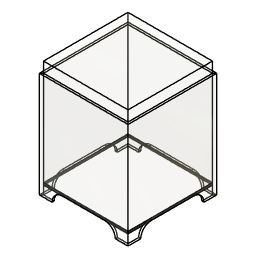
cube_fusion_model (Autodesk Fusion 360 design; units mm, degrees)
Autodesk Fusion 360 part; units mm, degrees
ref_plane "WorkPlane1" through (0, 0, 2) normal (0, 0, 1) x (1, 0, 0)
sketch "Sketch1" plane through (0, 0, 2) normal (0, 0, 1) x (1, 0, 0)
  line L0 (42.1, 42.1) -> (-42.1, 42.1)
  line L1 (-42.1, 42.1) -> (-42.1, -42.1)
  line L2 (-42.1, -42.1) -> (42.1, -42.1)
  line L3 (42.1, -42.1) -> (42.1, 42.1)
  line L4 (40, 40) -> (-40, 40)
  line L5 (-40, 40) -> (-40, -40)
  line L6 (-40, -40) -> (40, -40)
  line L7 (40, -40) -> (40, 40)
  line L8 (40, 40) -> (-40, -40) construction
  line L9 (-40, 40) -> (40, -40) construction
  line L10 (-40.1, 40.1) -> (-40.1, -40.1)
  line L11 (-40.1, -40.1) -> (40.1, -40.1)
  line L12 (40.1, -40.1) -> (40.1, 40.1)
  line L13 (40.1, 40.1) -> (-40.1, 40.1)
  line L14 (40.1, 40.1) -> (42.1, 42.1)
  line L15 (-40.1, 40.1) -> (-42.1, 42.1)
  line L16 (-40.1, -40.1) -> (-42.1, -42.1)
  line L17 (42.1, -42.1) -> (40.1, -40.1)
  dimension "d3" = 80
  dimension "d4" = 80
  dimension "d15" = -2
  dimension "d23" = 0.1
  dimension "d24" = 0.1
  dimension "d25" = 0.1
  dimension "d26" = 0.1
  constraint horizontal L0
  constraint perpendicular L0 L1
  constraint parallel L0 L2
  constraint parallel L1 L3
  constraint horizontal L4
  constraint perpendicular L4 L5
  constraint parallel L4 L6
  constraint parallel L5 L7
  constraint coincident L8 origin
  constraint coincident L9 origin
  measures "d3" distance of L5.end L6.end
  measures "d4" distance of L4.end L5.end
  measures "d23" distance of L6 L11
  measures "d24" distance of L5 L10
  measures "d25" distance of L4 L13
  measures "d26" distance of L7 L12
extrude "Extrude6" add sketch "Sketch1" against normal blind 2 contours L10 L11 L12 L13 makes body 1
extrude "Extrude7" add sketch "Sketch1" along normal blind 100 separate body contours L10 L11 L12 L13 | L4 L5 L6 L7 makes body 2
sketch "Sketch2" plane through (0, 40.1, 0) normal (0, 1, 0) x (-1, 0, 0)
  line L0 (42.1, 102) -> (-42.1, 102)
  line L1 (-42.1, 102) -> (-42.1, 2)
  line L2 (-42.1, 2) -> (42.1, 2)
  line L3 (42.1, 2) -> (42.1, 102)
  line L4 (20, 12) -> (-20, 12)
  line L5 (-20, 12) -> (-20, -8)
  line L6 (-20, -8) -> (20, -8)
  line L7 (20, -8) -> (20, 12)
  line L8 (20, 12) -> (-20, -8) construction
  line L9 (-20, 12) -> (20, -8) construction
  circle A0 centre (-20, 2) radius 10
  circle A1 centre (20, 2) radius 10
  line L10 (-40.1, 2) -> (40.1, 2)
  line L11 (40.1, 2) -> (40.1, 102)
  line L12 (40.1, 102) -> (-40.1, 102)
  line L13 (-40.1, 102) -> (-40.1, 2)
  point P0 (0, 2)
  dimension "d27" = 40
  dimension "d28" = 20
  constraint horizontal L4
  constraint perpendicular L4 L5
  constraint parallel L4 L6
  constraint parallel L5 L7
  constraint coincident L8 P0
  constraint coincident L9 P0
  constraint midpoint L2 P0
  constraint midpoint L5 A0.centre
  constraint coincident L4.end A0
  constraint midpoint L7 A1.centre
  constraint coincident L4.start A1
  measures "d27" distance of L5.end L6.end
  measures "d28" distance of L4.end L5.end
extrude "Extrude10" add sketch "Sketch1" along normal blind 100 separate body contours L0 L13 L14 L15 makes body 3
extrude "Extrude11" cut sketch "Sketch2" along normal blind 10 contours L2 L7 A1 L10 | L2 L5 A0 L10 | L2 L7 A1 L10 | L2 L4 A0 A1 L10 | L2 L5 A0 L10 picked at (20.4744, 8.6327) picked at (-26.6327, 2.4744) picked at (17.6762, 8.2304) picked at (-19.5256, 8.6327) bodies 3
pattern_circular "C-Pattern1" count 4 over 360 about axis through (0, 0, 1.75) along (0, 0, 1) of bodies 3 makes body 4 at (-42.1, -6.6667, 72) makes body 5 at (6.6667, -42.1, 72) makes body 6 at (42.1, 6.6667, 72)
move_body "Move1" bodies 1 to x (1, 0, 0) y (0, 1, 0) z (0, 0, 1) at (0, 0, 10)
move_body "Move2" bodies 2 to x (1, 0, 0) y (0, 1, 0) z (0, 0, 1) at (0, 0, 10)
